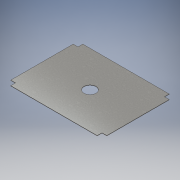
# Autodesk Inventor part: FrameSheetLaserViewport
Saved by Autodesk Inventor 2016 (Build 200138000, 138)
## iProperties
Created: 2015-08-02
Part Number: FrameSheetLaserViewport
Material: Steel, Galvanized
Document SubType Name: Sheet Metal
Designer: myhome
Density: 7.85 g/cm^3
Sheet Metal Rule: Default_mm
Appearance: Galvanized
Author: myhome
Autodesk Inventor part; units mm, degrees
ref_plane "YZ Plane" through (0, 0, 0) normal (1, 0, 0) x (0, 1, 0)
ref_plane "XZ Plane" through (0, 0, 0) normal (0, 1, 0) x (-1, 0, 0)
ref_plane "XY Plane" through (0, 0, 0) normal (0, 0, 1) x (1, 0, 0)
sketch "Sketch4" plane through (0, 0, 0) normal (0, 0, 1) x (1, 0, 0)
  line L0 (0, 0) -> (400, 0)
  line L1 (400, 0) -> (400, 300)
  line L2 (400, 300) -> (0, 300)
  line L3 (0, 300) -> (0, 0)
  dimension "d9" = 400
  dimension "d10" = 300
  measures "d9" distance of L1.end L2.end
  measures "d10" distance of L0.end L1.end
extrude "Plate2" add sketch "Sketch4" along normal blind 1.214
sketch "Sketch6" plane through (0, 0, 0) normal (0, 0, 1) x (1, 0, 0)
  line L0 (400, 0) -> (0, 0) projected
  line L1 (0, 300) -> (0, 0) projected
  circle A0 centre (200, 150) radius 25
  dimension "d13" = 50
  constraints: 1 centre point
  measures "d13" diameter of A0
extrude "Cut3" cut sketch "Sketch6" along normal blind 1.214
sketch "Sketch7" plane through (0, 0, 0) normal (0, 0, 1) x (1, 0, 0)
  line L0 (0, 0) -> (20, 0)
  line L1 (20, 0) -> (20, 20)
  line L2 (20, 20) -> (0, 20)
  line L3 (0, 20) -> (0, 0)
  dimension "d16" = 20
  dimension "d17" = 20
  constraints: 8 end point, 2 parallel, 1 horizontal, 1 perpendicular
  measures "d16" distance of L2.end L1.end
  measures "d17" distance of L0.end L1.end
extrude "Cut4" cut sketch "Sketch7" along normal blind 1.214
sketch "Sketch8" plane through (0, 0, 0) normal (0, 0, 1) x (1, 0, 0)
  line L0 (400, 0) -> (400, 300) projected
  line L1 (400, 0) -> (380, 0)
  line L2 (380, 0) -> (380, 20)
  line L3 (380, 20) -> (400, 20)
  line L4 (400, 20) -> (400, 0)
  line L5 (400, 300) -> (380, 300)
  line L6 (380, 300) -> (380, 280)
  line L7 (380, 280) -> (400, 280)
  line L8 (400, 280) -> (400, 300)
  line L9 (400, 300) -> (0, 300) projected
  line L10 (0, 300) -> (20, 300)
  line L11 (20, 300) -> (20, 280)
  line L12 (20, 280) -> (0, 280)
  line L13 (0, 280) -> (0, 300)
  point P0 (0, 0)
  dimension "d20" = 20
  dimension "d21" = 20
  dimension "d22" = 20
  dimension "d23" = 20
  dimension "d24" = 20
  dimension "d25" = 20
  constraints: 24 end point, 6 parallel, 3 horizontal, 3 perpendicular
  measures "d20" distance of L2.end L3.end
  measures "d21" distance of L1.end L2.end
  measures "d22" distance of L7.end L6.end
  measures "d23" distance of L5.end L6.end
  measures "d24" distance of L11.end L12.end
  measures "d25" distance of L10.end L11.end
extrude "Cut5" cut sketch "Sketch8" along normal blind 1.214
equation "\"d14\" = Thickness"
equation "\"d18\" = Thickness"
equation "\"d26\" = Thickness"
equation "\"BendRadius\" = Thickness"
equation "\"BendReliefWidth\" = Thickness"
equation "\"BendReliefDepth\" = 0.5 * Thickness"
equation "\"CornerReliefSize\" = 4 * Thickness"
equation "\"MinimumRemnant\" = 2 * Thickness"
equation "\"TransitionRadius\" = BendRadius"
equation "\"JacobiRadiusSize\" = BendRadius"
equation "\"GapSize\" = Thickness"
equation "\"d2\" = BendRadius"
equation "\"d11\" = BendRadius"
equation "\"Thickness\" = 1.214"
body "Solid2"
